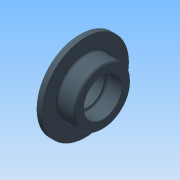
# Autodesk Inventor part: CoverInput
Saved by Autodesk Inventor 2020.1 (Build 241239000, 239)
## iProperties
Shininess: 64.0
Length Units: 11269
Angle Units: 11279
Time Units: 11290
Mass Units: 11283
Length Display Precision: 3
Angle Display Precision: 2
Compacted: True
Part Number: CoverInput
Document SubType Name: Modeling
Created: 2003-11-06
Designer: ales
Manufacturer: Standard
Standards Organization: Custom
Material: Generic
Density: 1 g/cm^3
Appearance: Blue Grey
Density: 0.0
Volumn: 0.0
Area: 0.0
PropertySet Name: Model Information
Control State: 0
Master: False
Checked Out: False
Author: ales
Autodesk Inventor part; units mm, degrees
ref_plane "YZ Plane" through (0, 0, 0) normal (1, 0, 0) x (0, 1, 0)
ref_plane "XZ Plane" through (0, 0, 0) normal (0, 1, 0) x (-1, 0, 0)
ref_plane "XY Plane" through (0, 0, 0) normal (0, 0, 1) x (1, 0, 0)
sketch "Sketch1" plane through (0, 0, 0) normal (0, 0, 1) x (1, 0, 0)
  line L0 (0, 0) -> (25.981, 0)
  line L1 (0, 16) -> (10, 16)
  line L2 (10, 16) -> (10, 18.5)
  line L3 (10, 18.5) -> (25, 18.5)
  line L4 (0, 22.5) -> (0, 16)
  line L5 (2, 22.5) -> (2, 42.5)
  line L6 (2, 42.5) -> (8, 42.5)
  line L7 (8, 42.5) -> (8, 27.5)
  line L8 (8, 27.5) -> (25, 27.5)
  line L9 (25, 27.5) -> (25, 18.5)
  line L10 (0, 22.5) -> (2, 22.5)
  dimension "d0" = 32
  dimension "d2" = 37
  dimension "d5" = 15
  dimension "d7" = 6
  dimension "d9" = 85
  dimension "d11" = 55
  dimension "d12" = 45
  dimension "d13" = 25
  dimension "d14" = 8
  constraints: 22 end point, 6 perpendicular, 1 horizontal, 1 parallel, 1 point on line, 1 vertical, 1 other
  measures "d0" diameter of L1 L0
  measures "d2" diameter of L3 L0
  measures "d5" distance of L2.end L3.end
  measures "d7" distance of L5.end L6.end
  measures "d9" diameter of L6 L0
  measures "d11" diameter of L8 L0
  measures "d12" diameter of L10 L0
  measures "d13" distance between parallel lines of L9 L4
  measures "d14" distance between parallel lines of L4 L7
revolve "Revolution1" add sketch "Sketch1" angle 360 about axis through (0, 0, 0) along (1, 0, 0)
fillet "Fillet1" radius 2 3 edges at (2, -22.5, 0) (10, -18.5, 0) (8, -27.5, 0)
chamfer "Chamfer2" distance 1 angle 45 2 edges at (25, -27.5, 0) (2, -42.5, 0)
body "Solid1"
